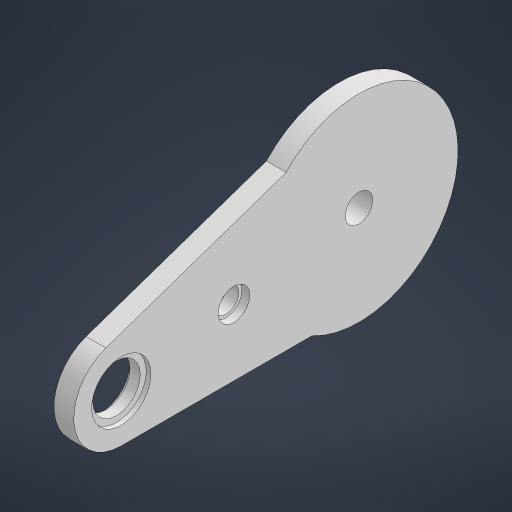
# Autodesk Inventor part: Main_Frame
Saved by Autodesk Inventor 2024.2 (Build 282272000, 272)
## iProperties
Created: 2024-03-05
Part Number: Main_Frame
Material: 一般
Document SubType Name: Modeling
Designer: Hanaoka
Density: 1 g/cm^3
Appearance: 既定
Author: Hanaoka
Autodesk Inventor part; units mm, degrees
ref_plane "YZ Plane" through (0, 0, 0) normal (1, 0, 0) x (0, 1, 0)
ref_plane "XZ Plane" through (0, 0, 0) normal (0, 1, 0) x (-1, 0, 0)
ref_plane "XY Plane" through (0, 0, 0) normal (0, 0, 1) x (1, 0, 0)
sketch "スケッチ1" plane through (0, 0, 0) normal (1, 0, 0) x (0, 1, 0)
  circle A0 centre (0, 0) radius 6
  circle A1 centre (5, -30) radius 11
  line L0 (-6, 0) -> (-6, -30)
  line L1 (5.6757, 1.9459) -> (15.4054, -26.4324)
  circle A2 centre (5, -30) radius 12.5
  circle A3 centre (0, 0) radius 3
  circle A4 centre (5, -30) radius 1.75
  line L2 (5, -30) -> (5, -41) construction
  circle A5 centre (0, 0) radius 4.5 construction
  circle A6 centre (5, -30) radius 2.5 construction
  line L3 (4.4778, 0.4463) -> (7.4877, -29.7521) construction
  line L4 (2.5664, -30.5723) -> (-4.3805, -1.0301) construction
  circle A7 centre (2.3696, -14.2177) radius 2
  circle A8 centre (2.3696, -14.2177) radius 1
  circle A9 centre (2.3696, -14.2177) radius 3.5522 construction
  line L5 (9.4297, -56.5784) -> (-3.4387, 20.6324) construction
  circle A10 centre (5, -30) radius 14 construction
  point P0 (-6, -24.0628)
  point P1 (13.4798, -20.8162)
  point P2 (15.9919, -30.4228)
  point P3 (-1.7415, -38.692)
  point P4 (13.8604, -21.1828)
  point P5 (-6.4987, -25.098)
  dimension "d0" = 12
  dimension "d1" = 22
  dimension "d2" = 30
  dimension "d3" = 25
  dimension "d4" = 6
  dimension "d5" = 3.5
  dimension "d21" = 9
  dimension "d22" = 5
  dimension "d23" = 2
  dimension "d24" = 4
  dimension "d35" = 28
  constraints: 13 point on circle, 12 end point, 11 centre point, 11 tangent, 9 coincident, 2 point on line, 2 vertical
  measures "d0" diameter of A0
  measures "d1" diameter of A1
  measures "d2" distance of L0.start L0.end
  measures "d3" diameter of A2
  measures "d4" diameter of A3
  measures "d5" diameter of A4
  measures "d21" diameter of A5
  measures "d22" diameter of A6
  measures "d23" diameter of A8
  measures "d24" diameter of A7
  measures "d35" diameter of A10
extrude "押し出し1" add sketch "スケッチ1" against normal blind 2.5 contours A0 | A0 L1 A2 L0 | A2 L0 A1 L1 | L1 A1 L0 A2 | A1 | A3 | A7 | A8
sketch "スケッチ2" plane through (-2.5, 0, 0) normal (-1, 0, 0) x (0, 0, 1)
  circle A0 centre (0, 0) radius 3.6
  circle A1 centre (0, 0) radius 3 projected
  dimension "d8" = 7.2
  constraints: 1 centre point, 1 coincident
  measures "d8" diameter of A0
extrude "押し出し2" cut sketch "スケッチ2" against normal blind 0.6
hole "穴1" at (0, 2.3696, -14.2177) direction (-1, 0, 0) diameter 3.2 end through all counterbore diameter 4 counterbore depth 1
hole "穴2" at (0, 0, 0) direction (-1, 0, 0) diameter 6 end through all counterbore diameter 7.5 counterbore depth 0.6
